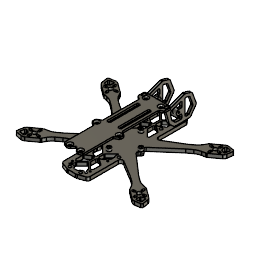
MerlynFPVFrame (Autodesk Fusion 360 design; units mm, degrees)
Autodesk Fusion 360 part; units mm, degrees
note: some values were not read from the file. Set by a fixed rule: which sketch regions a step uses.
(part 1 of 3)
sketch "Sketch1" plane through (0, 0, 0) normal (0, 0, 1) x (1, 0, 0)
  line L0 (15, 60) -> (-15, -60) construction
  line L1 (-15, 60) -> (15, -60) construction
  line L2 (20, 0) -> (2.5, 0)
  line L3 (0, 2.5) -> (0, 20)
  circle A0 centre (59, 43) radius 2.25
  line L4 (59, 43) -> (58.3414, 38.8013)
  line L5 (57.3535, 38.9563) -> (57.0668, 37.1287)
  arc A1 (57.0668, 37.1287) -> (59.0426, 36.8187) centre (58.0547, 36.9737) ccw
  line L6 (59.0426, 36.8187) -> (59.3293, 38.6464)
  arc A2 (59.3293, 38.6464) -> (57.3535, 38.9563) centre (58.3414, 38.8013) ccw
  line L7 (58.3414, 38.8013) -> (58.0547, 36.9737) construction
  arc A3 (59.4281, 38.6309) -> (57.2547, 38.9718) centre (58.3414, 38.8013) ccw
  line L8 (57.2547, 38.9718) -> (56.968, 37.1442)
  arc A4 (56.968, 37.1442) -> (59.1414, 36.8032) centre (58.0547, 36.9737) ccw
  line L9 (59.1414, 36.8032) -> (59.4281, 38.6309)
  arc A5 (64.8558, 40.968) -> (65.1968, 43.1414) centre (65.0263, 42.0547) ccw
  line L10 (65.1968, 43.1414) -> (63.3691, 43.4281)
  arc A6 (63.3691, 43.4281) -> (63.0282, 41.2547) centre (63.1987, 42.3414) ccw
  line L11 (63.0282, 41.2547) -> (64.8558, 40.968)
  arc A7 (61.032, 48.8558) -> (58.8586, 49.1968) centre (59.9453, 49.0263) ccw
  line L12 (58.8586, 49.1968) -> (58.5719, 47.3691)
  arc A8 (58.5719, 47.3691) -> (60.7453, 47.0282) centre (59.6586, 47.1987) ccw
  line L13 (60.7453, 47.0282) -> (61.032, 48.8558)
  arc A9 (53.1442, 45.032) -> (52.8032, 42.8586) centre (52.9737, 43.9453) ccw
  line L14 (52.8032, 42.8586) -> (54.6309, 42.5719)
  arc A10 (54.6309, 42.5719) -> (54.9718, 44.7453) centre (54.8013, 43.6586) ccw
  line L15 (54.9718, 44.7453) -> (53.1442, 45.032)
  line L16 (58.0547, 36.9737) -> (65.0263, 42.0547)
  line L17 (68.581, 41.6303) -> (58.4131, 34.2198)
  line L18 (50.4618, 45.1297) -> (60.6297, 52.5402)
  line L19 (59, 43) -> (62.9757, 37.545)
  line L20 (59, 43) -> (55.0243, 48.455)
  line L21 (70.3762, 44.5696) -> (71.3342, 50.6769)
  line L22 (63.9775, 53.3492) -> (70.0847, 52.3912)
  line L23 (49.7459, 44.3181) -> (47.8072, 40.8084)
  line L24 (57.4213, 33.7868) -> (53.4866, 33.0159)
  line L25 (43.3688, 35.7766) -> (38.0643, 31.9107)
  line L26 (47.3374, 30.3313) -> (42.033, 26.4653)
  line L27 (38.0643, 31.9107) -> (18.7908, 20.291)
  line L28 (42.033, 26.4653) -> (18.153, 5.6444)
  line L29 (68.1327, 45.1089) -> (68.783, 49.255)
  line L30 (63.804, 51.0483) -> (67.9501, 50.3979)
  line L31 (66.7394, 44.3498) -> (63.6069, 45.7389)
  line L32 (63.0179, 46.547) -> (62.6547, 49.9543)
  arc A11 (71.3342, 50.6769) -> (70.0847, 52.3912) centre (69.8523, 50.9093) ccw
  arc A12 (63.9775, 53.3492) -> (60.6297, 52.5402) centre (63.2801, 48.9036) ccw
  arc A13 (68.581, 41.6303) -> (70.3762, 44.5696) centre (65.9305, 45.2669) ccw
  arc A14 (57.4213, 33.7868) -> (58.4131, 34.2198) centre (56.9406, 36.2401) ccw
  arc A15 (50.4618, 45.1297) -> (49.7459, 44.3181) centre (51.9342, 43.1093) ccw
  arc A16 (53.4866, 33.0159) -> (47.3374, 30.3313) centre (56.4667, 17.8051) ccw
  arc A17 (43.3688, 35.7766) -> (47.8072, 40.8084) centre (34.2395, 48.3029) ccw
  arc A18 (63.0179, 46.547) -> (63.6069, 45.7389) centre (64.0123, 46.653) ccw
  arc A19 (63.804, 51.0483) -> (62.6547, 49.9543) centre (63.649, 50.0604) ccw
  arc A20 (68.783, 49.255) -> (67.9501, 50.3979) centre (67.7951, 49.41) ccw
  arc A21 (66.7394, 44.3498) -> (68.1327, 45.1089) centre (67.1447, 45.2639) ccw
  line L33 (38.0643, -31.9107) -> (18.7908, -20.291)
  line L34 (42.033, -26.4653) -> (18.153, -5.6444)
  line L35 (47.3374, -30.3313) -> (42.033, -26.4653)
  line L36 (43.3688, -35.7766) -> (38.0643, -31.9107)
  arc A22 (47.3374, -30.3313) -> (53.4866, -33.0159) centre (56.4667, -17.8051) ccw
  arc A23 (47.8072, -40.8084) -> (43.3688, -35.7766) centre (34.2395, -48.3029) ccw
  line L37 (57.4213, -33.7868) -> (53.4866, -33.0159)
  line L38 (49.7459, -44.3181) -> (47.8072, -40.8084)
  arc A24 (58.4131, -34.2198) -> (57.4213, -33.7868) centre (56.9406, -36.2401) ccw
  arc A25 (49.7459, -44.3181) -> (50.4618, -45.1297) centre (51.9342, -43.1093) ccw
  line L39 (50.4618, -45.1297) -> (60.6297, -52.5402)
  line L40 (68.581, -41.6303) -> (58.4131, -34.2198)
  arc A26 (70.3762, -44.5696) -> (68.581, -41.6303) centre (65.9305, -45.2669) ccw
  arc A27 (60.6297, -52.5402) -> (63.9775, -53.3492) centre (63.2801, -48.9036) ccw
  line L41 (63.9775, -53.3492) -> (70.0847, -52.3912)
  line L42 (70.3762, -44.5696) -> (71.3342, -50.6769)
  arc A28 (70.0847, -52.3912) -> (71.3342, -50.6769) centre (69.8523, -50.9093) ccw
  line L43 (63.804, -51.0483) -> (67.9501, -50.3979)
  arc A29 (62.6547, -49.9543) -> (63.804, -51.0483) centre (63.649, -50.0604) ccw
  line L44 (63.0179, -46.547) -> (62.6547, -49.9543)
  arc A30 (63.6069, -45.7389) -> (63.0179, -46.547) centre (64.0123, -46.653) ccw
  line L45 (66.7394, -44.3498) -> (63.6069, -45.7389)
  arc A31 (68.1327, -45.1089) -> (66.7394, -44.3498) centre (67.1447, -45.2639) ccw
  line L46 (68.1327, -45.1089) -> (68.783, -49.255)
  arc A32 (67.9501, -50.3979) -> (68.783, -49.255) centre (67.7951, -49.41) ccw
  line L47 (52.8032, -42.8586) -> (54.6309, -42.5719)
  arc A33 (54.9718, -44.7453) -> (54.6309, -42.5719) centre (54.8013, -43.6586) ccw
  line L48 (54.9718, -44.7453) -> (53.1442, -45.032)
  arc A34 (52.8032, -42.8586) -> (53.1442, -45.032) centre (52.9737, -43.9453) ccw
  arc A35 (60.7453, -47.0282) -> (58.5719, -47.3691) centre (59.6586, -47.1987) ccw
  line L49 (60.7453, -47.0282) -> (61.032, -48.8558)
  arc A36 (58.8586, -49.1968) -> (61.032, -48.8558) centre (59.9453, -49.0263) ccw
  line L50 (58.8586, -49.1968) -> (58.5719, -47.3691)
  line L51 (63.0282, -41.2547) -> (64.8558, -40.968)
  arc A37 (63.0282, -41.2547) -> (63.3691, -43.4281) centre (63.1987, -42.3414) ccw
  line L52 (65.1968, -43.1414) -> (63.3691, -43.4281)
  arc A38 (65.1968, -43.1414) -> (64.8558, -40.968) centre (65.0263, -42.0547) ccw
  circle A39 centre (59, -43) radius 2.25
  arc A40 (57.2547, -38.9718) -> (59.4281, -38.6309) centre (58.3414, -38.8013) ccw
  arc A41 (59.1414, -36.8032) -> (56.968, -37.1442) centre (58.0547, -36.9737) ccw
  line L53 (59.1414, -36.8032) -> (59.4281, -38.6309)
  line L54 (57.2547, -38.9718) -> (56.968, -37.1442)
  line L55 (-50.4618, 45.1297) -> (-60.6297, 52.5402)
  line L56 (-52.8032, 42.8586) -> (-54.6309, 42.5719)
  line L57 (-49.7459, 44.3181) -> (-47.8072, 40.8084)
  arc A42 (-53.4866, -33.0159) -> (-47.3374, -30.3313) centre (-56.4667, -17.8051) ccw
  line L58 (-63.0179, -46.547) -> (-62.6547, -49.9543)
  arc A43 (-52.8032, 42.8586) -> (-53.1442, 45.032) centre (-52.9737, 43.9453) ccw
  line L59 (-38.0643, -31.9107) -> (-18.7908, -20.291)
  arc A44 (-54.9718, 44.7453) -> (-54.6309, 42.5719) centre (-54.8013, 43.6586) ccw
  line L60 (-63.9775, -53.3492) -> (-70.0847, -52.3912)
  line L61 (-57.4213, -33.7868) -> (-53.4866, -33.0159)
  line L62 (-42.033, -26.4653) -> (-18.153, -5.6444)
  arc A45 (-68.783, -49.255) -> (-67.9501, -50.3979) centre (-67.7951, -49.41) ccw
  arc A46 (-47.8072, 40.8084) -> (-43.3688, 35.7766) centre (-34.2395, 48.3029) ccw
  arc A47 (-56.968, -37.1442) -> (-59.1414, -36.8032) centre (-58.0547, -36.9737) ccw
  line L63 (-54.9718, 44.7453) -> (-53.1442, 45.032)
  arc A48 (-49.7459, 44.3181) -> (-50.4618, 45.1297) centre (-51.9342, 43.1093) ccw
  line L64 (-52.8032, -42.8586) -> (-54.6309, -42.5719)
  arc A49 (-71.3342, -50.6769) -> (-70.0847, -52.3912) centre (-69.8523, -50.9093) ccw
  line L65 (-43.3688, 35.7766) -> (-38.0643, 31.9107)
  circle A50 centre (-59, 43) radius 2.25
  line L66 (-70.3762, 44.5696) -> (-71.3342, 50.6769)
  line L67 (-50.4618, -45.1297) -> (-60.6297, -52.5402)
  arc A51 (-57.4213, -33.7868) -> (-58.4131, -34.2198) centre (-56.9406, -36.2401) ccw
  circle A52 centre (-59, -43) radius 2.25
  arc A53 (-68.1327, 45.1089) -> (-66.7394, 44.3498) centre (-67.1447, 45.2639) ccw
  line L68 (-68.581, -41.6303) -> (-58.4131, -34.2198)
  line L69 (-66.7394, 44.3498) -> (-63.6069, 45.7389)
  arc A54 (-59.4281, -38.6309) -> (-57.2547, -38.9718) centre (-58.3414, -38.8013) ccw
  line L70 (-59.1414, 36.8032) -> (-59.4281, 38.6309)
  line L71 (-57.2547, -38.9718) -> (-56.968, -37.1442)
  arc A55 (-63.0179, -46.547) -> (-63.6069, -45.7389) centre (-64.0123, -46.653) ccw
  arc A56 (-54.6309, -42.5719) -> (-54.9718, -44.7453) centre (-54.8013, -43.6586) ccw
  line L72 (-60.7453, -47.0282) -> (-61.032, -48.8558)
  line L73 (-63.804, -51.0483) -> (-67.9501, -50.3979)
  arc A57 (-66.7394, -44.3498) -> (-68.1327, -45.1089) centre (-67.1447, -45.2639) ccw
  arc A58 (-58.5719, -47.3691) -> (-60.7453, -47.0282) centre (-59.6586, -47.1987) ccw
  arc A59 (-53.1442, -45.032) -> (-52.8032, -42.8586) centre (-52.9737, -43.9453) ccw
  line L74 (-57.4213, 33.7868) -> (-53.4866, 33.0159)
  line L75 (-47.3374, -30.3313) -> (-42.033, -26.4653)
  line L76 (-49.7459, -44.3181) -> (-47.8072, -40.8084)
  arc A60 (-43.3688, -35.7766) -> (-47.8072, -40.8084) centre (-34.2395, -48.3029) ccw
  line L77 (-43.3688, -35.7766) -> (-38.0643, -31.9107)
  arc A61 (-50.4618, -45.1297) -> (-49.7459, -44.3181) centre (-51.9342, -43.1093) ccw
  line L78 (-65.1968, -43.1414) -> (-63.3691, -43.4281)
  line L79 (-58.8586, -49.1968) -> (-58.5719, -47.3691)
  arc A62 (-47.3374, 30.3313) -> (-53.4866, 33.0159) centre (-56.4667, 17.8051) ccw
  arc A63 (-63.3691, -43.4281) -> (-63.0282, -41.2547) centre (-63.1987, -42.3414) ccw
  line L80 (-70.3762, -44.5696) -> (-71.3342, -50.6769)
  arc A64 (-68.581, -41.6303) -> (-70.3762, -44.5696) centre (-65.9305, -45.2669) ccw
  arc A65 (-64.8558, -40.968) -> (-65.1968, -43.1414) centre (-65.0263, -42.0547) ccw
  line L81 (-63.0282, -41.2547) -> (-64.8558, -40.968)
  arc A66 (-61.032, -48.8558) -> (-58.8586, -49.1968) centre (-59.9453, -49.0263) ccw
  arc A67 (-63.804, -51.0483) -> (-62.6547, -49.9543) centre (-63.649, -50.0604) ccw
  line L82 (-38.0643, 31.9107) -> (-18.7908, 20.291)
  line L83 (-59.1414, -36.8032) -> (-59.4281, -38.6309)
  arc A68 (-63.9775, -53.3492) -> (-60.6297, -52.5402) centre (-63.2801, -48.9036) ccw
  line L84 (-68.1327, -45.1089) -> (-68.783, -49.255)
  line L85 (-66.7394, -44.3498) -> (-63.6069, -45.7389)
  line L86 (-54.9718, -44.7453) -> (-53.1442, -45.032)
  line L87 (-63.0179, 46.547) -> (-62.6547, 49.9543)
  line L88 (-60.7453, 47.0282) -> (-61.032, 48.8558)
  arc A69 (-58.4131, 34.2198) -> (-57.4213, 33.7868) centre (-56.9406, 36.2401) ccw
  arc A70 (-57.2547, 38.9718) -> (-59.4281, 38.6309) centre (-58.3414, 38.8013) ccw
  arc A71 (-63.6069, 45.7389) -> (-63.0179, 46.547) centre (-64.0123, 46.653) ccw
  line L89 (-58.8586, 49.1968) -> (-58.5719, 47.3691)
  line L90 (-65.1968, 43.1414) -> (-63.3691, 43.4281)
  arc A72 (-60.6297, 52.5402) -> (-63.9775, 53.3492) centre (-63.2801, 48.9036) ccw
  arc A73 (-59.1414, 36.8032) -> (-56.968, 37.1442) centre (-58.0547, 36.9737) ccw
  line L91 (-63.9775, 53.3492) -> (-70.0847, 52.3912)
  line L92 (-63.804, 51.0483) -> (-67.9501, 50.3979)
  arc A74 (-60.7453, 47.0282) -> (-58.5719, 47.3691) centre (-59.6586, 47.1987) ccw
  line L93 (-68.581, 41.6303) -> (-58.4131, 34.2198)
  arc A75 (-70.3762, 44.5696) -> (-68.581, 41.6303) centre (-65.9305, 45.2669) ccw
  arc A76 (-58.8586, 49.1968) -> (-61.032, 48.8558) centre (-59.9453, 49.0263) ccw
  arc A77 (-67.9501, 50.3979) -> (-68.783, 49.255) centre (-67.7951, 49.41) ccw
  line L94 (-68.1327, 45.1089) -> (-68.783, 49.255)
  arc A78 (-65.1968, 43.1414) -> (-64.8558, 40.968) centre (-65.0263, 42.0547) ccw
  line L95 (-63.0282, 41.2547) -> (-64.8558, 40.968)
  arc A79 (-63.0282, 41.2547) -> (-63.3691, 43.4281) centre (-63.1987, 42.3414) ccw
  arc A80 (-62.6547, 49.9543) -> (-63.804, 51.0483) centre (-63.649, 50.0604) ccw
  arc A81 (-70.0847, 52.3912) -> (-71.3342, 50.6769) centre (-69.8523, 50.9093) ccw
  line L96 (-57.2547, 38.9718) -> (-56.968, 37.1442)
  line L97 (-42.033, 26.4653) -> (-18.153, 5.6444)
  line L98 (-47.3374, 30.3313) -> (-42.033, 26.4653)
  line L99 (-19.7635, -1.7678) -> (-18.0781, -3.4531)
  line L100 (-19.7635, 1.7678) -> (-18.0781, 3.4531)
  line L101 (18.0781, 3.4531) -> (19.7635, 1.7678)
  line L102 (18.0781, -3.4531) -> (19.7635, -1.7678)
  arc A82 (-18.0781, 3.4531) -> (-18.153, 5.6444) centre (-19.1387, 4.5138) ccw
  arc A83 (-18.153, -5.6444) -> (-18.0781, -3.4531) centre (-19.1387, -4.5138) ccw
  arc A84 (18.0781, -3.4531) -> (18.153, -5.6444) centre (19.1387, -4.5138) ccw
  arc A85 (18.153, 5.6444) -> (18.0781, 3.4531) centre (19.1387, 4.5138) ccw
  arc A86 (-15, -22.432) -> (-18.7908, -20.291) centre (-17.5, -22.432) ccw
  arc A87 (18.7908, -20.291) -> (15, -22.432) centre (17.5, -22.432) ccw
  arc A88 (-18.7908, 20.291) -> (-15, 22.432) centre (-17.5, 22.432) ccw
  arc A89 (15, 22.432) -> (18.7908, 20.291) centre (17.5, 22.432) ccw
  circle A90 centre (-59, -43) radius 38.1
  circle A91 centre (-59, 43) radius 38.1
  circle A92 centre (59, 43) radius 38.1
  circle A93 centre (59, -43) radius 38.1
  line L103 (0, 60) -> (-4.1184, 60)
  line L104 (0, 60) -> (4.1184, 60)
  line L105 (-5.8285, 59.6985) -> (-13.0261, 57.0788)
  line L106 (5.8285, 59.6985) -> (13.0261, 57.0788)
  line L107 (-15, 22.432) -> (-15, 54.2597)
  line L108 (15, 54.2597) -> (15, 22.432)
  line L109 (-10, 46.7051) -> (-10, 37.6399)
  line L110 (-8.2929, 47.4122) -> (-1.2929, 40.4122)
  line L111 (-10, 49.1193) -> (2.6802, 49.1193) construction
  line L112 (-9.5736, 36.8207) -> (-4.2583, 33.0989)
  line L113 (-10, 37.1193) -> (-1.9899, 37.1193) construction
  line L114 (-3.6847, 32.918) -> (-2, 32.918)
  line L115 (-1, 33.918) -> (-1, 39.7051)
  arc A94 (-8.2929, 47.4122) -> (-10, 46.7051) centre (-9, 46.7051) ccw
  arc A95 (-10, 37.6399) -> (-9.5736, 36.8207) centre (-9, 37.6399) ccw
  arc A96 (-1, 39.7051) -> (-1.2929, 40.4122) centre (-2, 39.7051) ccw
  arc A97 (-2, 32.918) -> (-1, 33.918) centre (-2, 33.918) ccw
  arc A98 (-4.2583, 33.0989) -> (-3.6847, 32.918) centre (-3.6847, 33.918) ccw
  line L116 (-3.6847, 31.4608) -> (-2, 31.4608)
  arc A99 (-1, 30.4608) -> (-2, 31.4608) centre (-2, 30.4608) ccw
  line L117 (-9.5736, 27.5581) -> (-4.2583, 31.2799)
  arc A100 (-3.6847, 31.4608) -> (-4.2583, 31.2799) centre (-3.6847, 30.4608) ccw
  line L118 (-1, 30.4608) -> (-1, 24.6738)
  line L119 (-8.2929, 16.9667) -> (-1.2929, 23.9667)
  arc A101 (-10, 17.6738) -> (-8.2929, 16.9667) centre (-9, 17.6738) ccw
  line L120 (-10, 17.6738) -> (-10, 26.739)
  arc A102 (-9.5736, 27.5581) -> (-10, 26.739) centre (-9, 26.739) ccw
  arc A103 (-1.2929, 23.9667) -> (-1, 24.6738) centre (-2, 24.6738) ccw
  line L121 (9.5736, 27.5581) -> (4.2583, 31.2799)
  arc A104 (10, 26.739) -> (9.5736, 27.5581) centre (9, 26.739) ccw
  line L122 (3.6847, 31.4608) -> (2, 31.4608)
  arc A105 (4.2583, 31.2799) -> (3.6847, 31.4608) centre (3.6847, 30.4608) ccw
  arc A106 (2, 31.4608) -> (1, 30.4608) centre (2, 30.4608) ccw
  line L123 (1, 30.4608) -> (1, 24.6738)
  line L124 (8.2929, 16.9667) -> (1.2929, 23.9667)
  arc A107 (1, 24.6738) -> (1.2929, 23.9667) centre (2, 24.6738) ccw
  arc A108 (8.2929, 16.9667) -> (10, 17.6738) centre (9, 17.6738) ccw
  line L125 (10, 17.6738) -> (10, 26.739)
  line L126 (10, 46.7051) -> (10, 37.6399)
  arc A109 (9.5736, 36.8207) -> (10, 37.6399) centre (9, 37.6399) ccw
  line L127 (9.5736, 36.8207) -> (4.2583, 33.0989)
  arc A110 (3.6847, 32.918) -> (4.2583, 33.0989) centre (3.6847, 33.918) ccw
  line L128 (3.6847, 32.918) -> (2, 32.918)
  arc A111 (1, 33.918) -> (2, 32.918) centre (2, 33.918) ccw
  line L129 (1, 33.918) -> (1, 39.7051)
  line L130 (8.2929, 47.4122) -> (1.2929, 40.4122)
  arc A112 (1.2929, 40.4122) -> (1, 39.7051) centre (2, 39.7051) ccw
  arc A113 (10, 46.7051) -> (8.2929, 47.4122) centre (9, 46.7051) ccw
  arc A114 (-13.0261, 57.0788) -> (-15, 54.2597) centre (-12, 54.2597) ccw
  arc A115 (15, 54.2597) -> (13.0261, 57.0788) centre (12, 54.2597) ccw
  arc A116 (-4.1184, 60) -> (-5.8285, 59.6985) centre (-4.1184, 55) ccw
  arc A117 (5.8285, 59.6985) -> (4.1184, 60) centre (4.1184, 55) ccw
  arc A118 (-19.7635, 1.7678) -> (-19.7635, -1.7678) centre (-17.9957, 0) ccw
  arc A119 (19.7635, -1.7678) -> (19.7635, 1.7678) centre (17.9957, 0) ccw
  line L131 (0, 55.5) -> (4.1184, 55.5)
  line L132 (10, 52.9799) -> (10, 51.5944)
  line L133 (9.7071, 50.8873) -> (0.7071, 41.8873)
  line L134 (10, 51.1801) -> (24.1421, 51.1801) construction
  line L135 (5.8285, 55.1985) -> (9.342, 53.9196)
  arc A120 (5.8285, 55.1985) -> (4.1184, 55.5) centre (4.1184, 50.5) ccw
  arc A121 (10, 52.9799) -> (9.342, 53.9196) centre (9, 52.9799) ccw
  arc A122 (9.7071, 50.8873) -> (10, 51.5944) centre (9, 51.5944) ccw
  line L136 (-9.7071, 50.8873) -> (-0.7071, 41.8873)
  line L137 (-10, 52.9799) -> (-10, 51.5944)
  arc A123 (-9.342, 53.9196) -> (-10, 52.9799) centre (-9, 52.9799) ccw
  arc A124 (-10, 51.5944) -> (-9.7071, 50.8873) centre (-9, 51.5944) ccw
  line L138 (-5.8285, 55.1985) -> (-9.342, 53.9196)
  line L139 (0, 55.5) -> (-4.1184, 55.5)
  arc A125 (-4.1184, 55.5) -> (-5.8285, 55.1985) centre (-4.1184, 50.5) ccw
  arc A126 (-0.7071, 41.8873) -> (0.7071, 41.8873) centre (0, 42.5944) ccw
  circle A127 centre (-10, -29.345) radius 1
  circle A128 centre (10, -29.345) radius 1
  circle A129 centre (-10, -49.345) radius 1
  circle A130 centre (10, -49.345) radius 1
  line L140 (-5.8285, -59.6985) -> (-13.0261, -57.0788)
  arc A131 (-9.5736, -36.8207) -> (-10, -37.6399) centre (-9, -37.6399) ccw
  line L141 (-1, -33.918) -> (-1, -39.7051)
  arc A132 (-5.8285, -59.6985) -> (-4.1184, -60) centre (-4.1184, -55) ccw
  line L142 (-9.5736, -36.8207) -> (-4.2583, -33.0989)
  arc A133 (4.2583, -33.0989) -> (3.6847, -32.918) centre (3.6847, -33.918) ccw
  arc A134 (-10, -52.9799) -> (-9.342, -53.9196) centre (-9, -52.9799) ccw
  arc A135 (-1, -33.918) -> (-2, -32.918) centre (-2, -33.918) ccw
  arc A136 (-1.2929, -40.4122) -> (-1, -39.7051) centre (-2, -39.7051) ccw
  arc A137 (-4.2583, -31.2799) -> (-3.6847, -31.4608) centre (-3.6847, -30.4608) ccw
  arc A138 (-3.6847, -32.918) -> (-4.2583, -33.0989) centre (-3.6847, -33.918) ccw
  line L143 (0, -60) -> (4.1184, -60)
  arc A139 (3.6847, -31.4608) -> (4.2583, -31.2799) centre (3.6847, -30.4608) ccw
  arc A140 (10, -37.6399) -> (9.5736, -36.8207) centre (9, -37.6399) ccw
  arc A141 (2, -32.918) -> (1, -33.918) centre (2, -33.918) ccw
  line L144 (-3.6847, -31.4608) -> (-2, -31.4608)
  arc A142 (13.0261, -57.0788) -> (15, -54.2597) centre (12, -54.2597) ccw
  arc A143 (1, -39.7051) -> (1.2929, -40.4122) centre (2, -39.7051) ccw
  line L145 (5.8285, -59.6985) -> (13.0261, -57.0788)
  line L146 (9.5736, -36.8207) -> (4.2583, -33.0989)
  arc A144 (9.342, -53.9196) -> (10, -52.9799) centre (9, -52.9799) ccw
  line L147 (1, -33.918) -> (1, -39.7051)
  line L148 (-3.6847, -32.918) -> (-2, -32.918)
  line L149 (-1, -30.4608) -> (-1, -24.6738)
  arc A145 (1, -30.4608) -> (2, -31.4608) centre (2, -30.4608) ccw
  arc A146 (0.7071, -41.8873) -> (-0.7071, -41.8873) centre (0, -42.5944) ccw
  line L150 (1, -30.4608) -> (1, -24.6738)
  arc A147 (-2, -31.4608) -> (-1, -30.4608) centre (-2, -30.4608) ccw
  arc A148 (4.1184, -60) -> (5.8285, -59.6985) centre (4.1184, -55) ccw
  line L151 (3.6847, -32.918) -> (2, -32.918)
  arc A149 (-15, -54.2597) -> (-13.0261, -57.0788) centre (-12, -54.2597) ccw
  line L152 (3.6847, -31.4608) -> (2, -31.4608)
  line L153 (0, -60) -> (-4.1184, -60)
  line L154 (-15, -22.432) -> (-15, -54.2597)
  line L155 (15, -54.2597) -> (15, -22.432)
  line L156 (-8.2929, -16.9667) -> (-1.2929, -23.9667)
  line L157 (8.2929, -16.9667) -> (1.2929, -23.9667)
  arc A150 (1.2929, -23.9667) -> (1, -24.6738) centre (2, -24.6738) ccw
  line L158 (0, -60) -> (0, -10)
  arc A151 (-8.5848, -46.6998) -> (-9.25, -46.4403) centre (-10, -49.345) ccw
  arc A152 (-9.5714, -52.3143) -> (-7.045, -48.8271) centre (-10, -49.345) ccw
  arc A153 (9.25, -46.4403) -> (8.5848, -46.6998) centre (10, -49.345) ccw
  arc A154 (7.045, -48.8271) -> (9.5714, -52.3143) centre (10, -49.345) ccw
  line L159 (-10, -45.472) -> (-10, -37.6399)
  line L160 (-7.4059, -46.5252) -> (-1.2929, -40.4122)
  line L161 (1.2929, -40.4122) -> (7.4059, -46.5252)
  line L162 (10, -45.472) -> (10, -37.6399)
  line L163 (-6.7672, -47.9473) -> (-0.7071, -41.8873)
  line L164 (0.7071, -41.8873) -> (6.7672, -47.9473)
  line L165 (-10, -52.8091) -> (-10, -52.9799)
  line L166 (10, -52.9799) -> (10, -52.8091)
  arc A155 (-9.5714, -52.3143) -> (-10, -52.8091) centre (-9.5, -52.8091) ccw
  arc A156 (10, -52.8091) -> (9.5714, -52.3143) centre (9.5, -52.8091) ccw
  arc A157 (-6.7672, -47.9473) -> (-7.045, -48.8271) centre (-6.0601, -48.6544) ccw
  arc A158 (7.045, -48.8271) -> (6.7672, -47.9473) centre (6.0601, -48.6544) ccw
  arc A159 (-8.5848, -46.6998) -> (-7.4059, -46.5252) centre (-8.113, -45.8181) ccw
  arc A160 (7.4059, -46.5252) -> (8.5848, -46.6998) centre (8.113, -45.8181) ccw
  arc A161 (9.25, -46.4403) -> (10, -45.472) centre (9, -45.472) ccw
  arc A162 (-10, -45.472) -> (-9.25, -46.4403) centre (-9, -45.472) ccw
  arc A163 (-1, -24.6738) -> (-1.2929, -23.9667) centre (-2, -24.6738) ccw
  arc A164 (-6.935, -28.9943) -> (-9.2448, -26.3539) centre (-10, -29.345) ccw
  arc A165 (9.2448, -26.3539) -> (6.935, -28.9943) centre (10, -29.345) ccw
  line L167 (-6.5151, -29.6997) -> (-4.2583, -31.2799)
  line L168 (4.2583, -31.2799) -> (6.5151, -29.6997)
  arc A166 (-6.935, -28.9943) -> (-6.5151, -29.6997) centre (-5.9415, -28.8805) ccw
  arc A167 (6.5151, -29.6997) -> (6.935, -28.9943) centre (5.9415, -28.8805) ccw
  arc A168 (-10, -25.3844) -> (-9.2448, -26.3539) centre (-9, -25.3844) ccw
  arc A169 (9.2448, -26.3539) -> (10, -25.3844) centre (9, -25.3844) ccw
  circle A170 centre (-18.0312, 0) radius 1.075
  circle A171 centre (18.0312, 0) radius 1.075
  circle A172 centre (0, -18.0312) radius 1.075
  circle A173 centre (0, 18.0312) radius 1.075
  line L169 (-18.0312, 0) -> (-15.7687, 0) construction
  line L170 (-19.1859, -2) -> (-16.8765, -2)
  line L171 (-16.8765, -2) -> (-15.7218, 0)
  line L172 (-15.7218, 0) -> (-16.8765, 2)
  line L173 (-16.8765, 2) -> (-19.1859, 2)
  line L174 (-19.1859, 2) -> (-20.3406, 0)
  line L175 (-20.3406, 0) -> (-19.1859, -2)
  line L176 (18.0312, 0) -> (20.358, 0) construction
  line L177 (20.3406, 0) -> (19.1859, 2)
  line L178 (19.1859, 2) -> (16.8765, 2)
  line L179 (16.8765, 2) -> (15.7218, 0)
  line L180 (15.7218, 0) -> (16.8765, -2)
  line L181 (16.8765, -2) -> (19.1859, -2)
  line L182 (19.1859, -2) -> (20.3406, 0)
  line L183 (0, 18.0312) -> (3.8028, 18.0312) construction
  line L184 (1.1547, 20.0312) -> (-1.1547, 20.0312)
  line L185 (-1.1547, 20.0312) -> (-2.3094, 18.0312)
  line L186 (-2.3094, 18.0312) -> (-1.1547, 16.0312)
  line L187 (-1.1547, 16.0312) -> (1.1547, 16.0312)
  line L188 (1.1547, 16.0312) -> (2.3094, 18.0312)
  line L189 (2.3094, 18.0312) -> (1.1547, 20.0312)
  line L190 (0, -18.0312) -> (4.1621, -18.0312) construction
  line L191 (2.3094, -18.0312) -> (1.1547, -16.0312)
  line L192 (1.1547, -16.0312) -> (-1.1547, -16.0312)
  line L193 (-1.1547, -16.0312) -> (-2.3094, -18.0312)
  line L194 (-2.3094, -18.0312) -> (-1.1547, -20.0312)
  line L195 (-1.1547, -20.0312) -> (1.1547, -20.0312)
  line L196 (1.1547, -20.0312) -> (2.3094, -18.0312)
  circle A174 centre (-6, -56) radius 1.575
  circle A175 centre (6, -56) radius 1.575
  circle A176 centre (-12.5, -19.2597) radius 1.575
  circle A177 centre (12.5, -19.2597) radius 1.575
  circle A178 centre (-12.5, -19.2597) radius 3
  circle A179 centre (12.5, -19.2597) radius 3
  circle A180 centre (-8.5, 32.168) radius 1.575
  circle A181 centre (8.5, 32.168) radius 1.575
  circle A182 centre (-8.5, 32.168) radius 3
  circle A183 centre (8.5, 32.168) radius 3
  circle A184 centre (6, -56) radius 3
  circle A185 centre (-6, -56) radius 3
  arc A186 (8.7144, -53.7905) -> (2.7002, -54.8333) centre (6, -56) ccw
  arc A187 (-2.7002, -54.8333) -> (-8.7144, -53.7905) centre (-6, -56) ccw
  line L197 (1.7574, -55.5) -> (-1.7574, -55.5)
  line L198 (-9.2732, -53.9447) -> (-9.342, -53.9196)
  line L199 (9.2732, -53.9447) -> (9.342, -53.9196)
  arc A188 (8.7144, -53.7905) -> (9.2732, -53.9447) centre (9.1022, -53.4748) ccw
  arc A189 (-9.2732, -53.9447) -> (-8.7144, -53.7905) centre (-9.1022, -53.4748) ccw
  arc A190 (1.7574, -55.5) -> (2.7002, -54.8333) centre (1.7574, -54.5) ccw
  arc A191 (-2.7002, -54.8333) -> (-1.7574, -55.5) centre (-1.7574, -54.5) ccw
  arc A192 (9.5099, -17.4405) -> (9.7778, -21.4596) centre (12.5, -19.2597) ccw
  arc A193 (-9.7778, -21.4596) -> (-9.5099, -17.4405) centre (-12.5, -19.2597) ccw
  arc A194 (9.1655, -16.6876) -> (8.2929, -16.9667) centre (9, -17.6738) ccw
  arc A195 (-8.2929, -16.9667) -> (-9.1655, -16.6876) centre (-9, -17.6738) ccw
  line L200 (10, -22.0881) -> (10, -25.3844)
  line L201 (-10, -22.0881) -> (-10, -25.3844)
  arc A196 (9.5099, -17.4405) -> (9.1655, -16.6876) centre (9.0827, -17.1807) ccw
  arc A197 (-9.1655, -16.6876) -> (-9.5099, -17.4405) centre (-9.0827, -17.1807) ccw
  arc A198 (10, -22.0881) -> (9.7778, -21.4596) centre (9, -22.0881) ccw
  arc A199 (-9.7778, -21.4596) -> (-10, -22.0881) centre (-9, -22.0881) ccw
  line L202 (10, -29.345) -> (14.9591, -29.345) construction
  line L203 (12.3094, -29.345) -> (11.1547, -27.345)
  line L204 (11.1547, -27.345) -> (8.8453, -27.345)
  line L205 (8.8453, -27.345) -> (7.6906, -29.345)
  line L206 (7.6906, -29.345) -> (8.8453, -31.345)
  line L207 (8.8453, -31.345) -> (11.1547, -31.345)
  line L208 (11.1547, -31.345) -> (12.3094, -29.345)
  line L209 (-10, -29.345) -> (-5.2547, -29.345) construction
  line L210 (-11.1547, -31.345) -> (-8.8453, -31.345)
  line L211 (-8.8453, -31.345) -> (-7.6906, -29.345)
  line L212 (-7.6906, -29.345) -> (-8.8453, -27.345)
  line L213 (-8.8453, -27.345) -> (-11.1547, -27.345)
  line L214 (-11.1547, -27.345) -> (-12.3094, -29.345)
  line L215 (-12.3094, -29.345) -> (-11.1547, -31.345)
  line L216 (10, -49.345) -> (14, -49.345) construction
  line L217 (-10, -49.345) -> (-5.0686, -49.345) construction
  line L218 (12.3094, -49.345) -> (11.1547, -47.345)
  line L219 (11.1547, -47.345) -> (8.8453, -47.345)
  line L220 (8.8453, -47.345) -> (7.6906, -49.345)
  line L221 (7.6906, -49.345) -> (8.8453, -51.345)
  line L222 (8.8453, -51.345) -> (11.1547, -51.345)
  line L223 (11.1547, -51.345) -> (12.3094, -49.345)
  line L224 (-11.1547, -51.345) -> (-8.8453, -51.345)
  line L225 (-8.8453, -51.345) -> (-7.6906, -49.345)
  line L226 (-7.6906, -49.345) -> (-8.8453, -47.345)
  line L227 (-8.8453, -47.345) -> (-11.1547, -47.345)
  line L228 (-11.1547, -47.345) -> (-12.3094, -49.345)
  line L229 (-12.3094, -49.345) -> (-11.1547, -51.345)
  point P0 (70.0873, 42.7281)
  point P1 (57.9652, 33.8933)
  point P2 (50.0139, 44.8033)
  point P3 (62.136, 53.638)
  point P4 (46.1458, 37.8005)
  point P5 (50.1144, 32.3552)
  point P6 (67.9307, 43.8215)
  point P7 (68.938, 50.2429)
  point P8 (62.5165, 51.2502)
  point P9 (-59.3293, 38.6464)
  point P10 (-67.9307, 43.8215)
  point P11 (-70.0873, 42.7281)
  point P12 (-62.5165, 51.2502)
  point P13 (-50.0139, 44.8033)
  point P14 (-68.938, 50.2429)
  point P15 (-58.0547, 36.9737)
  point P16 (-57.9652, 33.8933)
  point P17 (-50.1144, 32.3552)
  point P18 (-46.1458, 37.8005)
  point P19 (-58.3414, 38.8013)
  point P20 (-58.0547, 36.9737)
  point P21 (-65.0263, 42.0547)
  point P22 (-62.136, 53.638)
  point P23 (-59, 43)
  point P24 (-62.9757, 37.545)
  point P25 (-57.3535, 38.9563)
  point P26 (-59.0426, 36.8187)
  point P27 (-57.0668, 37.1287)
  point P28 (-58.3414, 38.8013)
  point P29 (-59, 43)
  point P30 (-5, 60)
  point P31 (5, 60)
  point P32 (-1, 40.1193)
  point P33 (-4, 32.918)
  point P34 (-1, 32.918)
  point P35 (5, 55.5)
  point P36 (10, 53.6801)
  point P37 (-4, -32.918)
  point P38 (-1, -40.1193)
  point P39 (-1.9899, -37.1193)
  point P40 (-2, -24.6738)
  point P41 (5, -55.5)
  point P42 (-15, -60)
  point P43 (10, -51.1801)
  point P44 (-5, -60)
  point P45 (-1, -32.918)
  point P46 (10, -53.6801)
  point P47 (5, -60)
  point P48 (2.6802, -49.1193)
  point P49 (-10, -37.1193)
  point P50 (15, -60)
  point P51 (-10, -49.1193)
  point P52 (-18.0312, 0)
  point P53 (18.0312, 0)
  point P54 (0, 18.0312)
  point P55 (0, -18.0312)
  point P56 (10, -29.345)
  point P57 (-10, -29.345)
  point P58 (10, -49.345)
  point P59 (-10, -49.345)
  dimension "d23" = 30
  dimension "d24" = 120
  dimension "d79" = 4.5
  dimension "d80" = 4.25
  dimension "d82" = 1.85
  dimension "d83" = 2
  dimension "d84" = 0.1
  dimension "d86" = 360
  dimension "d87" = 15
  dimension "d88" = 13.5
  dimension "d89" = 15
  dimension "d92" = 135
  dimension "d93" = 135
  dimension "d97" = 8
  dimension "d98" = 8
  dimension "d99" = 155
  dimension "d100" = 155
  dimension "d101" = 10
  dimension "d102" = 10
  dimension "d103" = 175
  dimension "d104" = 175
  dimension "d106" = 6.5
  dimension "d107" = 6.5
  dimension "d109" = 75
  dimension "d110" = 75
  dimension "d111" = 1.5
  dimension "d112" = 4.5
  dimension "d113" = 2.5
  dimension "d114" = 2.5
  dimension "d115" = 15.5
  dimension "d116" = 1
  dimension "d117" = 1.5
  dimension "d118" = 1.5
  dimension "d119" = 2.5
  dimension "d120" = 76.2
  dimension "d121" = 76.2
  dimension "d122" = 76.2
  dimension "d123" = 76.2
  dimension "d125" = 5
  dimension "d126" = 5
  dimension "d138" = 12
  dimension "d141" = 5
  dimension "d143" = 45
  dimension "d144" = 9
  dimension "d145" = 35
  dimension "d146" = 6
  dimension "d147" = 3
  dimension "d156" = 1
  dimension "d160" = 3
  dimension "d161" = 5
  dimension "d162" = 2.5
  dimension "d163" = 5
  dimension "d166" = 2.5
  dimension "d167" = 135
  dimension "d168" = 5
  dimension "d169" = 1
  dimension "d170" = 1
  dimension "d172" = 20
  dimension "d173" = 20
  dimension "d174" = 20
  dimension "d175" = 2
  dimension "d176" = 2
  dimension "d177" = 2
  dimension "d178" = 2
  dimension "d179" = 3
  dimension "d180" = 3
  dimension "d181" = 3
  dimension "d182" = 3
  dimension "d183" = 0.5
  dimension "d184" = 1
  dimension "d185" = 1
  dimension "d186" = 1
  dimension "d189" = 2.15
  dimension "d190" = 2.15
  dimension "d191" = 2.15
  dimension "d192" = 2.15
  dimension "d193" = 90
  dimension "d194" = 90
  dimension "d195" = 90
  dimension "d196" = 25.5
  dimension "d198" = 2
  dimension "d200" = 2
  dimension "d202" = 2
  dimension "d204" = 2
  dimension "d205" = 3.15
  dimension "d206" = 3.15
  dimension "d207" = 6
  dimension "d208" = 6
  dimension "d211" = 3.15
  dimension "d212" = 3.15
  dimension "d213" = 2.5
  dimension "d214" = 2.5
  dimension "d215" = 35
  dimension "d216" = 35
  dimension "d217" = 6
  dimension "d218" = 6
  dimension "d219" = 3.15
  dimension "d220" = 3.15
  dimension "d221" = 6
  dimension "d222" = 6
  dimension "d223" = 6.5
  dimension "d224" = 6.5
  dimension "d225" = 0.75
  dimension "d226" = 0.75
  dimension "d229" = 6
  dimension "d230" = 6
  dimension "d231" = 3.5
  dimension "d232" = 3.5
  dimension "d233" = 0.5
  dimension "d234" = 1
  dimension "d235" = 3.5
  dimension "d236" = 3.5
  dimension "d237" = 0.5
  dimension "d238" = 1
  dimension "d240" = 2
  dimension "d242" = 2
  dimension "d246" = 2
  dimension "d247" = 2
  constraint coincident L0 origin
  constraint coincident L1 origin
  constraint coincident A0.centre L4.start
  constraint tangent L5 A1
  constraint tangent A1 L6
  constraint parallel L5 L6
  constraint tangent L6 A2
  constraint tangent L5 A2
  constraint parallel L4 L7
  constraint coincident L4.end A2.centre
  constraint coincident A1.centre L7.end
  constraint coincident A5.centre L16.end
  constraint parallel L16 L17
  constraint coincident L17 L19.end
  constraint perpendicular L17 L19
  constraint coincident L18 L20.end
  constraint perpendicular L18 L20
  constraint equal L19 L20
  constraint perpendicular L21 L22
  constraint parallel L18 L25
  constraint parallel L17 L26
  constraint tangent L21 A11
  constraint tangent L22 A11
  constraint coincident P3 L18
  constraint coincident P3 L22
  constraint tangent L18 A12
  constraint tangent L22 A12
  constraint coincident P0 L17
  constraint coincident P0 L21
  constraint tangent L17 A13
  constraint tangent L21 A13
  constraint equal A12 A13
  constraint coincident P1 L17
  constraint coincident P1 L24
  constraint tangent L17 A14
  constraint tangent L24 A14
  constraint coincident P2 L18
  constraint coincident P2 L23
  constraint tangent L18 A15
  constraint tangent L23 A15
  constraint coincident P5 L24
  constraint coincident P5 L26
  constraint tangent L24 A16
  constraint tangent L26 A16
  constraint coincident P4 L23
  constraint coincident P4 L25
  constraint tangent L23 A17
  constraint tangent L25 A17
  constraint equal A16 A17
  constraint tangent L31 A18
  constraint tangent L32 A18
  constraint coincident P8 L30
  constraint coincident P8 L32
  constraint tangent L30 A19
  constraint tangent L32 A19
  constraint equal A18 A19
  constraint coincident P7 L29
  constraint coincident P7 L30
  constraint tangent L29 A20
  constraint tangent L30 A20
  constraint equal A18 A20
  constraint coincident P6 L29
  constraint coincident P6 L31
  constraint tangent L29 A21
  constraint tangent L31 A21
  constraint equal A18 A21
  constraint symmetric L2 A0 A39
  constraint symmetric L2 A3.end A40.start
  constraint symmetric L2 A3.start A40.end
  constraint symmetric L2 A3 A40
  constraint symmetric L2 L8.end A41.end
  constraint symmetric L2 A4.end A41.start
  constraint symmetric L2 A4 A41
  constraint symmetric L2 A5.start L51.end
  constraint symmetric L2 A5.end L52.start
  constraint symmetric L2 A5 A38
  constraint symmetric L2 L10.end A37.end
  constraint symmetric L2 A6.end L51.start
  constraint symmetric L2 A6 A37
  constraint symmetric L2 A7.start L49.end
  constraint symmetric L2 A7.end A36.start
  constraint symmetric L2 A7 A36
  constraint symmetric L2 L12.end A35.end
  constraint symmetric L2 A8.end A35.start
  constraint symmetric L2 A8 A35
  constraint symmetric L2 A9.start L48.end
  constraint symmetric L2 A9.end L47.start
  constraint symmetric L2 A9 A34
  constraint symmetric L2 L14.end L47.end
  constraint symmetric L2 A10.end A33.start
  constraint symmetric L2 A10 A33
  constraint symmetric L2 L25.end L33.start
  constraint symmetric L2 L26.end L34.start
  constraint symmetric L2 L21.end L42.end
  constraint symmetric L2 L22.end L41.end
  constraint symmetric L2 A11 A28
  constraint symmetric L2 L18.end L39.end
  constraint symmetric L2 L22.start A27.end
  constraint symmetric L2 A12 A27
  constraint symmetric L2 L17.start L40.start
  constraint symmetric L2 L21.start A26.start
  constraint symmetric L2 A13 A26
  constraint symmetric L2 L17.end A24.start
  constraint symmetric L2 L24.start L37.start
  constraint symmetric L2 A14 A24
  constraint symmetric L2 L18.start A25.end
  constraint symmetric L2 L23.start L38.start
  constraint symmetric L2 A15 A25
  constraint symmetric L2 L24.end A22.end
  constraint symmetric L2 L26.start L35.start
  constraint symmetric L2 A16 A22
  constraint symmetric L2 L23.end A23.start
  constraint symmetric L2 L25.start L36.start
  constraint symmetric L2 A17 A23
  constraint symmetric L2 L31.end A30.start
  constraint symmetric L2 L32.start L44.start
  constraint symmetric L2 A18 A30
  constraint symmetric L2 L30.start L43.start
  constraint symmetric L2 L32.end A29.start
  constraint symmetric L2 A19 A29
  constraint symmetric L2 L29.end L46.end
  constraint symmetric L2 L30.end L43.end
  constraint symmetric L2 A20 A32
  constraint symmetric L2 L29.start A31.start
  constraint symmetric L2 L31.start L45.start
  constraint symmetric L2 A21 A31
  constraint symmetric L3 A0 A50
  constraint symmetric L3 A0.centre P29
  constraint symmetric L3 L4.end P28
  constraint symmetric L3 L5.start P25
  constraint symmetric L3 L5.end P27
  constraint symmetric L3 A1.end P26
  constraint symmetric L3 L6.end P9
  constraint symmetric L3 A1.centre P15
  constraint symmetric L3 A3.end A70.start
  constraint symmetric L3 A3.start L70.end
  constraint symmetric L3 A3 A70
  constraint symmetric L3 L8.end A73.end
  constraint symmetric L3 A4.end L70.start
  constraint symmetric L3 A4 A73
  constraint symmetric L3 A5.start A78.end
  constraint symmetric L3 A5.end L90.start
  constraint symmetric L3 A5 A78
  constraint symmetric L3 L10.end L90.end
  constraint symmetric L3 A6.end L95.start
  constraint symmetric L3 A6 A79
  constraint symmetric L3 A7.start L88.end
  constraint symmetric L3 A7.end L89.start
  constraint symmetric L3 A7 A76
  constraint symmetric L3 L12.end L89.end
  constraint symmetric L3 A8.end L88.start
  constraint symmetric L3 A8 A74
  constraint symmetric L3 A9.start A43.end
  constraint symmetric L3 A9.end L56.start
  constraint symmetric L3 A9 A43
  constraint symmetric L3 L14.end L56.end
  constraint symmetric L3 A10.end A44.start
  constraint symmetric L3 A10 A44
  constraint symmetric L3 A1.centre P20
  constraint symmetric L3 A5.centre P21
  constraint symmetric L3 P0 P11
  constraint symmetric L3 P1 P16
  constraint symmetric L3 P2 P13
  constraint symmetric L3 P3 P22
  constraint symmetric L3 L19.end P24
  constraint symmetric L3 P4 P18
  constraint symmetric L3 P5 P17
  constraint symmetric L3 L25.end L65.end
  constraint symmetric L3 L26.end L97.start
  constraint symmetric L3 P6 P10
  constraint symmetric L3 P7 P14
  constraint symmetric L3 P8 P12
  constraint symmetric L3 L21.end L66.end
  constraint symmetric L3 L22.end L91.end
  constraint symmetric L3 A11 A81
  constraint symmetric L3 L18.end L55.end
  constraint symmetric L3 L22.start A72.end
  constraint symmetric L3 A12 A72
  constraint symmetric L3 L17.start L93.start
  constraint symmetric L3 L21.start L66.start
  constraint symmetric L3 A13 A75
  constraint symmetric L3 L17.end A69.start
  constraint symmetric L3 L24.start L74.start
  constraint symmetric L3 A14 A69
  constraint symmetric L3 L18.start L55.start
  constraint symmetric L3 L23.start L57.start
  constraint symmetric L3 A15 A48
  constraint symmetric L3 L24.end L74.end
  constraint symmetric L3 L26.start A62.start
  constraint symmetric L3 A16 A62
  constraint symmetric L3 L23.end L57.end
  constraint symmetric L3 L25.start A46.end
  constraint symmetric L3 A17 A46
  constraint symmetric L3 L31.end L69.end
  constraint symmetric L3 L32.start L87.start
  constraint symmetric L3 A18 A71
  constraint symmetric L3 L30.start L92.start
  constraint symmetric L3 L32.end L87.end
  constraint symmetric L3 A19 A80
  constraint symmetric L3 L29.end A77.end
  constraint symmetric L3 L30.end L92.end
  constraint symmetric L3 A20 A77
  constraint symmetric L3 L29.start A53.start
  constraint symmetric L3 L31.start A53.end
  constraint symmetric L3 A21 A53
  constraint symmetric L3 L33.start L59.start
  constraint symmetric L3 L34.start L62.start
  constraint symmetric L3 L35.start A42.end
  constraint symmetric L3 L36.start A60.start
  constraint symmetric L3 A22.end A42.start
  constraint symmetric L3 A22 A42
  constraint symmetric L3 A23.start L76.end
  constraint symmetric L3 A23 A60
  constraint symmetric L3 L37.start L61.start
  constraint symmetric L3 L38.start L76.start
  constraint symmetric L3 A24.start A51.end
  constraint symmetric L3 A24 A51
  constraint symmetric L3 A25.end L67.start
  constraint symmetric L3 A25 A61
  constraint symmetric L3 L39.end L67.end
  constraint symmetric L3 L40.start L68.start
  constraint symmetric L3 A26.start L80.start
  constraint symmetric L3 A26 A64
  constraint symmetric L3 A27.end L60.start
  constraint symmetric L3 A27 A68
  constraint symmetric L3 L41.end L60.end
  constraint symmetric L3 L42.end A49.start
  constraint symmetric L3 A28 A49
  constraint symmetric L3 L43.start L73.start
  constraint symmetric L3 L43.end A45.end
  constraint symmetric L3 A29.start L58.end
  constraint symmetric L3 A29 A67
  constraint symmetric L3 L44.start L58.start
  constraint symmetric L3 A30.start A55.end
  constraint symmetric L3 A30 A55
  constraint symmetric L3 L45.start A57.start
  constraint symmetric L3 A31.start A57.end
  constraint symmetric L3 A31 A57
  constraint symmetric L3 L46.end A45.start
  constraint symmetric L3 A32 A45
  constraint symmetric L3 L47.start L64.start
  constraint symmetric L3 L47.end L64.end
  constraint symmetric L3 A33.start A56.end
  constraint symmetric L3 A33 A56
  constraint symmetric L3 L48.end A59.start
  constraint symmetric L3 A34 A59
  constraint symmetric L3 A35.end A58.start
  constraint symmetric L3 A35.start L72.start
  constraint symmetric L3 A35 A58
  constraint symmetric L3 L49.end L72.end
  constraint symmetric L3 A36.start L79.start
  constraint symmetric L3 A36 A66
  constraint symmetric L3 L51.start A63.end
  constraint symmetric L3 L51.end A65.start
  constraint symmetric L3 A37.end L78.end
  constraint symmetric L3 A37 A63
  constraint symmetric L3 L52.start L78.start
  constraint symmetric L3 A38 A65
  constraint symmetric L3 A39 A52
  constraint symmetric L3 A40.end A54.start
  constraint symmetric L3 A40.start A54.end
  constraint symmetric L3 A40 A54
  constraint symmetric L3 A41.end A47.start
  constraint symmetric L3 A41.start A47.end
  constraint symmetric L3 A41 A47
  constraint perpendicular L99 L100
  constraint perpendicular L101 L102
  constraint tangent L97 A82
  constraint tangent L100 A82
  constraint tangent L62 A83
  constraint tangent L99 A83
  constraint equal A82 A83
  constraint tangent L34 A84
  constraint tangent L102 A84
  constraint tangent L28 A85
  constraint tangent L101 A85
  constraint equal A84 A85
  constraint tangent L59 A86
  constraint tangent L33 A87
  constraint equal A86 A87
  constraint tangent L82 A88
  constraint equal A86 A88
  constraint tangent L27 A89
  constraint equal A86 A89
  constraint concentric A52 A90
  constraint coincident P29 P23
  constraint concentric A0 A92
  constraint concentric A39 A93
  constraint tangent A88 L107
  constraint tangent A89 L108
  constraint horizontal L111
  constraint horizontal L113
  constraint horizontal L114
  constraint coincident L111.start L109
  constraint coincident L111.start L110
  constraint tangent L109 A94
  constraint tangent L110 A94
  constraint coincident L113.start L112
  constraint coincident L113.start L109
  constraint tangent L112 A95
  constraint tangent L109 A95
  constraint equal A94 A95
  constraint coincident P32 L110
  constraint coincident P32 L115
  constraint tangent L110 A96
  constraint tangent L115 A96
  constraint equal A94 A96
  constraint coincident P34 L114
  constraint coincident P34 L115
  constraint tangent L114 A97
  constraint tangent L115 A97
  constraint equal A94 A97
  constraint coincident P33 L112
  constraint coincident P33 L114
  constraint tangent L112 A98
  constraint tangent L114 A98
  constraint equal A94 A98
  constraint tangent L105 A114
  constraint tangent L107 A114
  constraint tangent L106 A115
  constraint tangent L108 A115
  constraint equal A114 A115
  constraint coincident P30 L103
  constraint coincident P30 L105
  constraint tangent L103 A116
  constraint tangent L105 A116
  constraint coincident P31 L104
  constraint coincident P31 L106
  constraint tangent L104 A117
  constraint tangent L106 A117
  constraint equal A116 A117
  constraint tangent L99 A118
  constraint tangent L100 A118
  constraint tangent L102 A119
  constraint tangent L101 A119
  constraint equal A118 A119
  constraint horizontal L134
  constraint coincident P35 L131
  constraint coincident P35 L135
  constraint tangent L131 A120
  constraint tangent L135 A120
  constraint coincident P36 L132
  constraint coincident P36 L135
  constraint tangent L132 A121
  constraint tangent L135 A121
  constraint coincident L134.start L133
  constraint coincident L134.start L132
  constraint tangent L133 A122
  constraint tangent L132 A122
  constraint equal A121 A122
  constraint tangent L136 A126
  constraint tangent L133 A126
  constraint perpendicular L143 L158
  constraint coincident P59 A129.centre
  constraint coincident P58 A130.centre
  constraint tangent A131 L159
  constraint tangent A136 L160
  constraint tangent A143 L161
  constraint tangent A140 L162
  constraint tangent A146 L163
  constraint tangent A146 L164
  constraint tangent A134 L165
  constraint tangent A144 L166
  constraint tangent A152 A155
  constraint tangent L165 A155
  constraint tangent A154 A156
  constraint tangent L166 A156
  constraint equal A155 A156
  constraint tangent A152 A157
  constraint tangent L163 A157
  constraint tangent A154 A158
  constraint tangent L164 A158
  constraint equal A157 A158
  constraint tangent A151 A159
  constraint tangent L160 A159
  constraint tangent A153 A160
  constraint tangent L161 A160
  constraint equal A159 A160
  constraint tangent A153 A161
  constraint tangent L162 A161
  constraint equal A159 A161
  constraint tangent A151 A162
  constraint tangent L159 A162
  constraint equal A159 A162
  constraint symmetric L150.end L158 L149.end
  constraint symmetric L157.end L158 L156.end
  constraint symmetric A150 L158 A163
  constraint coincident P57 A127.centre
  constraint coincident P56 A128.centre
  constraint tangent A137 L167
  constraint tangent A139 L168
  constraint tangent A164 A166
  constraint tangent L167 A166
  constraint tangent A165 A167
  constraint tangent L168 A167
  constraint equal A166 A167
  constraint tangent A164 A168
  constraint equal A166 A168
  constraint tangent A165 A169
  constraint equal A166 A169
  constraint coincident L158 P55
  constraint horizontal L169
  constraint coincident P52 A170.centre
  constraint horizontal L176
  constraint coincident P53 A171.centre
  constraint horizontal L183
  constraint coincident P54 A173.centre
  constraint horizontal L190
  constraint coincident P55 A172.centre
  constraint concentric A176 A178
  constraint concentric A177 A179
  constraint concentric A180 A182
  constraint concentric A181 A183
  constraint concentric A175 A184
  constraint concentric A174 A185
  constraint coincident A175.centre A184.centre
  constraint coincident A174.centre A185.centre
  constraint horizontal L197
  constraint tangent A134 L198
  constraint tangent A144 L199
  constraint tangent A186 A188
  constraint tangent L199 A188
  constraint tangent A187 A189
  constraint tangent L198 A189
  constraint equal A188 A189
  constraint tangent A186 A190
  constraint tangent L197 A190
  constraint tangent A187 A191
  constraint tangent L197 A191
  constraint equal A190 A191
  constraint coincident A177.centre A179.centre
  constraint coincident A176.centre A178.centre
  constraint tangent A169 L200
  constraint tangent A168 L201
  constraint tangent A192 A196
  constraint tangent A194 A196
  constraint tangent A193 A197
  constraint tangent A195 A197
  constraint equal A196 A197
  constraint tangent A192 A198
  constraint tangent L200 A198
  constraint tangent A193 A199
  constraint tangent L201 A199
  constraint equal A198 A199
  constraint horizontal L202
  constraint horizontal L209
  constraint horizontal L216
  constraint horizontal L217
  measures "d23" distance of P42 P50
  measures "d24" distance of L1.start P42
  measures "d79" diameter of A0
  measures "d80" distance of A0.centre L4.end
  measures "d82" distance of L4.end A1.centre
  measures "d83" diameter of A1
  measures "d87" distance of P0 P1
  measures "d88" distance of P1 P2
  measures "d89" distance of P2 P3
  measures "d92" angle of L17 L21
  measures "d93" angle of L18 L22
  measures "d97" distance of P2 P4
  measures "d98" distance of P1 P5
  measures "d99" angle of L18 L23
  measures "d100" angle of L17 L24
  measures "d101" distance of P4 L25.end
  measures "d102" distance of P5 L26.end
  measures "d103" angle of L25 L27
  measures "d104" angle of L26 L28
  measures "d106" distance of P7 P8
  measures "d107" distance of P6 P7
  measures "d109" angle of L29 L31
  measures "d110" angle of L30 L32
  measures "d111" radius of A11
  measures "d112" radius of A12
  measures "d113" radius of A14
  measures "d114" radius of A15
  measures "d115" radius of A16
  measures "d116" radius of A18
  measures "d117" radius of A82
  measures "d118" radius of A84
  measures "d119" radius of A86
  measures "d120" diameter of A90
  measures "d121" diameter of A91
  measures "d122" diameter of A92
  measures "d123" diameter of A93
  measures "d125" distance of L103.start P30
  measures "d126" distance of L103.start P31
  measures "d138" distance of L111.start L113.start
  measures "d141" distance of L107 L109
  measures "d143" angle of L110 L111
  measures "d144" distance of L109 P32
  measures "d145" angle of L112 L113
  measures "d146" distance of L109 P33
  measures "d147" distance of P33 P34
  measures "d156" radius of A94
  measures "d160" radius of A114
  measures "d161" radius of A116
  measures "d162" radius of A118
  measures "d163" distance of L131.start P35
  measures "d166" distance of P36 L134.start
  measures "d167" angle of L133 L134
  measures "d168" radius of A120
  measures "d169" radius of A121
  measures "d170" radius of A126
  measures "d172" distance of P57 P59
  measures "d173" distance of P59 P58
  measures "d174" distance of P56 P58
  measures "d175" diameter of A127
  measures "d176" diameter of A129
  measures "d177" diameter of A130
  measures "d178" diameter of A128
  measures "d179" radius of A152
  measures "d180" radius of A151
  measures "d181" radius of A154
  measures "d182" radius of A153
  measures "d183" radius of A155
  measures "d184" radius of A157
  measures "d185" radius of A159
  measures "d186" radius of A166
  measures "d189" diameter of A170
  measures "d190" diameter of A171
  measures "d191" diameter of A172
  measures "d192" diameter of A173
  measures "d193" angle of origin P52 P54